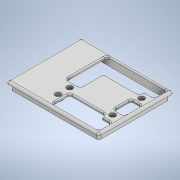
# Autodesk Inventor part: Lokk
Saved by Autodesk Inventor 2022 (Build 260153000, 153)
## iProperties
Created: 2021-08-17
Part Number: Lokk
Material: Generic
Document SubType Name: Modeling
Designer: Bruker
Density: 1 g/cm^3
Appearance: Default
Author: Bruker
Autodesk Inventor part; units mm, degrees
ref_plane "YZ Plane" through (0, 0, 0) normal (1, 0, 0) x (0, 1, 0)
ref_plane "XZ Plane" through (0, 0, 0) normal (0, 1, 0) x (-1, 0, 0)
ref_plane "XY Plane" through (0, 0, 0) normal (0, 0, 1) x (1, 0, 0)
sketch "Sketch1" plane through (0, 0, 0) normal (0, 1, 0) x (-1, 0, 0)
  line L0 (0, 0) -> (80, 0)
  line L1 (80, 0) -> (80, -65)
  line L2 (80, -65) -> (0, -65)
  line L3 (0, -65) -> (0, 0)
  dimension "d0" = 65
  dimension "d1" = 80
  constraints: 8 end point, 2 parallel, 1 horizontal, 1 perpendicular
  measures "d0" distance of L0.end L1.end
  measures "d1" distance of L1.end L2.end
extrude "Grunnflate" add sketch "Sketch1" along normal blind 2
sketch "Sketch2" plane through (0, 0, 0) normal (0, -1, 0) x (1, 0, 0)
  line L0 (-2, -2) -> (-78, -2)
  line L1 (-78, -2) -> (-78, -63)
  line L2 (-78, -63) -> (-2, -63)
  line L3 (-2, -63) -> (-2, -2)
  line L4 (0, -65) -> (-80, -65) projected
  line L5 (-80, -65) -> (-80, 0) projected
  line L6 (-80, 0) -> (0, 0) projected
  line L7 (0, 0) -> (0, -65) projected
  line L8 (-3, -3) -> (-77, -3)
  line L9 (-77, -3) -> (-77, -62)
  line L10 (-77, -62) -> (-3, -62)
  line L11 (-3, -62) -> (-3, -3)
  dimension "d4" = 2
  dimension "d5" = 2
  dimension "d6" = 2
  dimension "d7" = 2
  dimension "d8" = 1
  dimension "d9" = 1
  dimension "d10" = 1
  dimension "d11" = 1
  constraints: 16 end point, 4 parallel, 2 horizontal, 2 perpendicular
  measures "d4" distance between parallel lines of L4 L2
  measures "d5" distance between parallel lines of L5 L1
  measures "d6" distance between parallel lines of L6 L0
  measures "d7" distance between parallel lines of L7 L3
  measures "d8" distance between parallel lines of L3 L11
  measures "d9" distance between parallel lines of L2 L10
  measures "d10" distance between parallel lines of L1 L9
  measures "d11" distance between parallel lines of L0 L8
extrude "Vegger" add sketch "Sketch2" along normal blind 5 contours L3 L2 L1 L0
sketch "Sketch3" plane through (0, 2, 0) normal (0, 1, 0) x (1, 0, 0)
  line L0 (-3, 3) -> (-77, 3)
  line L1 (-77, 3) -> (-77, 62)
  line L2 (-77, 62) -> (-3, 62)
  line L3 (-3, 62) -> (-3, 3)
  line L4 (-80, 65) -> (-80, 0) projected
  line L5 (0, 65) -> (-80, 65) projected
  line L6 (0, 0) -> (0, 65) projected
  line L7 (-80, 0) -> (0, 0) projected
  line L8 (-55, 3) -> (-3, 3)
  line L9 (-3, 3) -> (-3, 62)
  line L10 (-3, 62) -> (-55, 62)
  line L11 (-55, 62) -> (-55, 3)
  line L12 (-55, 3) -> (-43, 3)
  line L13 (-43, 3) -> (-43, 27)
  line L14 (-43, 27) -> (-55, 27)
  line L15 (-55, 27) -> (-55, 3)
  line L16 (-43, 18) -> (-12, 18)
  line L17 (-12, 18) -> (-12, 47)
  line L18 (-12, 47) -> (-43, 47)
  line L19 (-43, 47) -> (-43, 18)
  line L20 (-12, 25) -> (-3, 25)
  line L21 (-3, 25) -> (-3, 14)
  line L22 (-3, 14) -> (-12, 14)
  line L23 (-12, 14) -> (-12, 25)
  line L24 (-12, 40) -> (-3, 40)
  line L25 (-3, 40) -> (-3, 51)
  line L26 (-3, 51) -> (-12, 51)
  line L27 (-12, 51) -> (-12, 40)
  point P0 (-12, 18)
  point P1 (-3, 40)
  point P2 (-3, 25)
  dimension "d14" = 3
  dimension "d15" = 3
  dimension "d16" = 3
  dimension "d17" = 3
  dimension "d18" = 52
  dimension "d19" = 0
  dimension "d20" = 0
  dimension "d21" = 0
  dimension "d22" = 34
  dimension "d23" = 0
  dimension "d24" = 24
  dimension "d25" = 0
  dimension "d26" = 15
  dimension "d27" = 15
  dimension "d28" = 9
  dimension "d29" = 0
  dimension "d30" = 0
  dimension "d31" = 22
  dimension "d32" = 11
  dimension "d33" = 0
  dimension "d34" = 22
  dimension "d35" = 11
  constraints: 48 end point, 12 parallel, 6 horizontal, 6 perpendicular, 2 point on line
  measures "d14" distance between parallel lines of L4 L1
  measures "d15" distance between parallel lines of L5 L2
  measures "d16" distance between parallel lines of L6 L3
  measures "d17" distance between parallel lines of L7 L0
  measures "d18" distance of L9.end L10.end
  measures "d19" distance between parallel lines of L3 L9
  measures "d20" distance between parallel lines of L2 L10
  measures "d21" distance between parallel lines of L0 L8
  measures "d22" distance between parallel lines of L1 L13
  measures "d23" distance between parallel lines of L11 L15
  measures "d24" distance of L12.end L13.end
  measures "d25" distance between parallel lines of L0 L12
  measures "d26" distance between parallel lines of L0 L16
  measures "d27" distance between parallel lines of L10 L18
  measures "d28" distance between parallel lines of L3 L17
  measures "d29" distance between parallel lines of L17 L23
  measures "d30" distance between parallel lines of L9 L21
  measures "d31" distance between parallel lines of L8 L20
  measures "d32" distance between parallel lines of L0 L22
  measures "d33" distance between parallel lines of L9 L25
  measures "d34" distance between parallel lines of L2 L24
  measures "d35" distance between parallel lines of L10 L26
extrude "Hull" cut sketch "Sketch3" against normal blind 2 contours L0 L13 L16 L23 L22 L3 | L20 L17 L24 L3 | L11 L2 L3 L26 L27 L18 L19 L14
fillet "Fillet1" radius 2 8 edges at (-2, -2.5, -2) (-78, -2.5, -2) (-2, -2.5, -63) (-78, -2.5, -63) (-3, -1.5, -62) (-3, -1.5, -3) (-77, -2.5, -62) (-77, -2.5, -3)
fillet "Fillet2" radius 2 4 edges at (-80, 1, 0) (-80, 1, -65) (0, 1, -65) (0, 1, 0)
fillet "Fillet3" radius 2 5 edges at (-43, 1, -3) (-3, 1, -14) (-12, 1, -14) (-12, 1, -18) (-43, 1, -18)
fillet "Fillet4" radius 2 7 edges at (-55, 1, -62) (-3, 1, -51) (-12, 1, -51) (-12, 1, -47) (-43, 1, -47) (-43, 1, -27) (-55, 1, -27)
fillet "Fillet5" radius 2 4 edges at (-12, 1, -40) (-3, 1, -40) (-3, 1, -25) (-12, 1, -25)
fillet "Fillet6" radius 2 8 edges at (-79.4142, 2, -64.4142) (-80, 2, -32.5) (-79.4142, 2, -0.5858) (-40, 2, 0) (-0.5858, 2, -0.5858) (0, 2, -32.5) (-0.5858, 2, -64.4142) (-40, 2, -65)
fillet "Fillet7" radius 1 34 edges at (-54.4144, 2, -61.4144) (-29.0003, 2, -62) (-3.5858, 2, -61.4142) (-3, 2, -56.4997) (-3.5856, 2, -51.5856) (-7.5, 2, -51) (-11.4144, 2, -50.4144) (-12.5856, 2, -47.5856) (-27.5, 2, -47) (-42.4144, 2, -46.4144) (-43, 2, -37) (-43.5856, 2, -27.5856) (-49, 2, -27) (-54.4144, 2, -27.5856) (-55, 2, -44.5) (-11.4142, 2, -39.4142) (-7.5, 2, -40) (-3.5858, 2, -39.4142) (-3, 2, -32.5) (-3.5858, 2, -25.5858) (-7.5, 2, -25) (-11.4142, 2, -25.5858) (-12, 2, -32.5) (-12.5856, 2, -17.4144) (-11.4144, 2, -14.5856) (-7.5, 2, -14) (-3.5856, 2, -13.4144) (-3, 2, -8.5003) (-3.5858, 2, -3.5858) (-23.0002, 2, -3) (-42.4144, 2, -3.5856) (-43, 2, -10.5) (-42.4144, 2, -17.4144) (-27.5, 2, -18)
sketch "Knapper Layout" plane through (0, 2, 0) normal (0, 1, 0) x (1, 0, 0)
  line L0 (-77, 3) -> (-3, 3)
  line L1 (-3, 3) -> (-3, 62)
  line L2 (-3, 62) -> (-77, 62)
  line L3 (-77, 62) -> (-77, 3)
  line L4 (-2, 65) -> (-78, 65) projected
  line L5 (0, 2) -> (0, 63) projected
  line L6 (-78, 0) -> (-2, 0) projected
  line L7 (-80, 63) -> (-80, 2) projected
  line L8 (-11, 17) -> (-5, 17)
  line L9 (-5, 17) -> (-5, 23)
  line L10 (-5, 23) -> (-11, 23)
  line L11 (-11, 23) -> (-11, 17)
  line L12 (-11, 42) -> (-5, 42)
  line L13 (-5, 42) -> (-5, 48)
  line L14 (-5, 48) -> (-11, 48)
  line L15 (-11, 48) -> (-11, 42)
  line L16 (-50, 9) -> (-44, 9)
  line L17 (-44, 9) -> (-44, 15)
  line L18 (-44, 15) -> (-50, 15)
  line L19 (-50, 15) -> (-50, 9)
  line L20 (-50, 19) -> (-44, 19)
  line L21 (-44, 19) -> (-44, 25)
  line L22 (-44, 25) -> (-50, 25)
  line L23 (-50, 25) -> (-50, 19)
  circle A0 centre (-47, 12) radius 2.5
  circle A1 centre (-47, 22) radius 2.5
  circle A2 centre (-8, 45) radius 2.5
  circle A3 centre (-8, 20) radius 2.5
  point P0 (0, 0)
  dimension "d45" = 3
  dimension "d46" = 3
  dimension "d47" = 3
  dimension "d48" = 3
  dimension "d49" = 20
  dimension "d50" = 14
  dimension "d51" = 20
  dimension "d52" = 14
  dimension "d53" = 8
  dimension "d54" = 8
  dimension "d55" = 2
  dimension "d56" = 2
  dimension "d57" = 33
  dimension "d58" = 33
  dimension "d59" = 6
  dimension "d60" = 6
  dimension "d61" = 4
  dimension "d62" = 6
  dimension "d63" = 6
  dimension "d64" = 6
  dimension "d65" = 5
  dimension "d67" = 5
  dimension "d68" = 5
  dimension "d69" = 5
  constraints: 40 end point, 10 parallel, 5 horizontal, 5 perpendicular, 4 centre point
  measures "d45" distance between parallel lines of L4 L2
  measures "d46" distance between parallel lines of L5 L1
  measures "d47" distance between parallel lines of L6 L0
  measures "d48" distance between parallel lines of L7 L3
  measures "d49" distance between parallel lines of L0 L10
  measures "d50" distance between parallel lines of L2 L14
  measures "d51" distance between parallel lines of L2 L12
  measures "d52" distance between parallel lines of L0 L8
  measures "d53" distance between parallel lines of L1 L11
  measures "d54" distance between parallel lines of L1 L15
  measures "d55" distance between parallel lines of L1 L13
  measures "d56" distance between parallel lines of L1 L9
  measures "d57" distance between parallel lines of L21 L3
  measures "d58" distance between parallel lines of L3 L17
  measures "d59" distance of L21.end L22.end
  measures "d60" distance of L17.end L18.end
  measures "d61" distance between parallel lines of L20 L18
  measures "d62" distance of L18.end L16.start
  measures "d63" distance of L22.end L20.start
  measures "d64" distance between parallel lines of L0 L16
  measures "d65" diameter of A2
  measures "d67" diameter of A3
  measures "d68" diameter of A0
  measures "d69" diameter of A1
extrude "Knappehull" cut sketch "Knapper Layout" against normal blind 9.75 contours A0 | A1 | A2 | A3
sketch "Sketch6" plane through (0, 0, 0) normal (0, -1, 0) x (1, 0, 0)
  circle A0 centre (-8, -45) radius 2.5 projected
  circle A1 centre (-8, -45) radius 3.5
  circle A2 centre (-8, -20) radius 2.5 projected
  circle A3 centre (-8, -20) radius 3.5
  circle A4 centre (-47, -22) radius 2.5 projected
  circle A5 centre (-47, -22) radius 3.5
  circle A6 centre (-47, -12) radius 2.5 projected
  circle A7 centre (-47, -12) radius 3.5
  point P0 (0, 0)
  dimension "d72" = 7
  dimension "d73" = 7
  dimension "d74" = 7
  dimension "d75" = 7
  constraints: 4 centre point, 4 coincident
  measures "d72" diameter of A7
  measures "d73" diameter of A5
  measures "d74" diameter of A1
  measures "d75" diameter of A3
extrude "Extrusion5" add sketch "Sketch6" along normal blind 1
sketch "Sketch7" plane through (-78, 0, -61) normal (-1, 0, 0) x (0, 0, 1)
  line L0 (59, -5) -> (57, -5) projected
  line L1 (32, 0) -> (16, 0) projected
  line L2 (57, -5) -> (16, -5)
  line L3 (16, -5) -> (16, 0)
  line L4 (16, 0) -> (57, 0)
  line L5 (57, 0) -> (57, -5)
  point P0 (61, 0)
  point P1 (32, 0)
  constraints: 8 end point, 2 parallel, 1 horizontal, 1 perpendicular
extrude "Extrusion6" cut sketch "Sketch7" against normal blind 2.5
body "Solid1"
